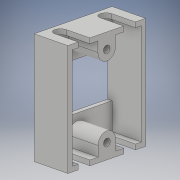
# Autodesk Inventor part: ssr-cover
Saved by Autodesk Inventor 2018 (Build 220112000, 112)
## iProperties
Created: 2020-01-09
Part Number: ssr-cover
Material: Generic
Document SubType Name: Modeling
Designer: Vinnie Caprarola
Density: 1 g/cm^3
Appearance: Default
Author: Vinnie Caprarola
Autodesk Inventor part; units mm, degrees
ref_plane "YZ Plane" through (0, 0, 0) normal (1, 0, 0) x (0, 1, 0)
sketch "Sketch1" plane through (0, 0, 0) normal (0, 0, 1) x (1, 0, 0)
  line L0 (0, 0) -> (45, 0)
  line L1 (45, 0) -> (45, 58)
  line L2 (45, 58) -> (0, 58)
  line L3 (0, 58) -> (0, 0)
  circle A0 centre (22.5, 53) radius 2.75
  circle A1 centre (22.5, 5) radius 2.75
  line L4 (19.75, 58) -> (19.75, 53)
  line L5 (25.25, 58) -> (25.25, 53)
  line L6 (0, 42) -> (45, 42)
  line L7 (45, 42) -> (45, 16)
  line L8 (45, 16) -> (0, 16)
  line L9 (0, 16) -> (0, 42)
  circle A2 centre (22.5, 53) radius 6
  circle A3 centre (22.5, 5) radius 6
  line L10 (16.5, 5) -> (16.5, -1)
  line L11 (28.5, 5) -> (28.5, -1)
  line L12 (16.5, 53) -> (16.5, 59)
  line L13 (28.5, 53) -> (28.5, 59)
  line L14 (-1, 59) -> (46, 59)
  line L15 (46, 59) -> (46, -1)
  line L16 (46, -1) -> (-1, -1)
  line L17 (-1, -1) -> (-1, 59)
  line L18 (49, 62) -> (-4, 62)
  line L19 (-4, 62) -> (-4, -4)
  line L20 (-4, -4) -> (49, -4)
  line L21 (49, -4) -> (49, 62)
  line L22 (28.5, 59) -> (16.5, 59)
  line L23 (28.5, -1) -> (16.5, -1)
  point P0 (22.5, 58)
  dimension "d0" = 45
  dimension "d1" = 58
  dimension "d2" = 5.5
  dimension "d3" = 5.5
  dimension "d4" = 5
  dimension "d5" = 5
  dimension "d6" = 26
  dimension "d7" = 16
  dimension "d8" = 12
  dimension "d9" = 12
  dimension "d10" = 1
  dimension "d11" = 3
  constraints: 48 end point, 10 parallel, 10 point on line, 6 perpendicular, 6 point on circle, 4 centre point, 4 tangent, 2 coincident, 2 horizontal, 2 vertical alignment, 1 collinear, 1 midpoint, 1 vertical, 6 other
  measures "d0" distance of L1.end L2.end
  measures "d1" distance of L0.end L1.end
  measures "d2" diameter of A0
  measures "d3" diameter of A1
  measures "d4" distance from line of A1.centre L0
  measures "d5" distance from line of A0.centre L2
  measures "d6" distance between parallel lines of L8 L6
  measures "d7" distance between parallel lines of L6 L2
  measures "d8" diameter of A2
  measures "d9" diameter of A3
  measures "d10" distance between parallel lines of L2 L14
  measures "d11" distance between parallel lines of L14 L18
extrude "Extrusion1" add sketch "Sketch1" along normal blind 10 contours L21 L20 L19 L18
sketch "Sketch2" plane through (0, 0, 10) normal (0, 0, 1) x (1, 0, 0)
  line L0 (-1, 59) -> (46, 59) projected
  line L1 (46, 59) -> (46, -1) projected
  line L2 (-1, 59) -> (46, 59)
  line L3 (46, 59) -> (46, 43)
  line L4 (46, 43) -> (-1, 43)
  line L5 (-1, 43) -> (-1, 59)
  line L6 (-1, -1) -> (-1, 59) projected
  line L7 (46, -1) -> (-1, -1)
  line L8 (-1, -1) -> (-1, 15)
  line L9 (-1, 15) -> (46, 15)
  line L10 (46, 15) -> (46, -1)
  point P0 (0, 0)
  dimension "d14" = 16
  dimension "d15" = 16
  constraints: 16 end point, 4 parallel, 2 horizontal, 2 perpendicular, 2 point on line
  measures "d14" distance of L2.end L3.end
  measures "d15" distance of L7.end L8.end
extrude "Extrusion2" add sketch "Sketch2" against normal blind 3 contours L0 L1 L4 L5 | L9 L1 L7 L6
sketch "Sketch3" plane through (0, 0, 0) normal (0, 0, -1) x (-1, 0, 0)
  arc A0 (-28.5, 53) -> (-16.5, 53) centre (-22.5, 53) ccw
  line L0 (-46, 59) -> (1, 59) projected
  line L1 (-28.5, 59) -> (-28.5, 53)
  line L2 (-16.5, 59) -> (-16.5, 53)
  line L3 (-16.5, 59) -> (-28.5, 59)
  point P0 (0, 0)
  dimension "d18" = 12
  constraints: 6 end point, 2 perpendicular, 2 point on circle, 2 point on line, 1 centre point, 1 coincident, 1 parallel
  measures "d18" diameter of A0
extrude "Extrusion3" add sketch "Sketch3" against normal up to surface (7 mm away)
ref_plane "Work Plane1" through (-4, 29, 0) normal (0, 1, 0) x (1, 0, 0)
mirror "Mirror1" about plane through (-4, 29, 0) normal (0, 1, 0) of "Extrusion3"
thicken "Thicken1" operation add thickness 13 both sides no extend neighbours yes toward (0, 0, -1) faces at (48, 39, 0)
sketch "Sketch4" plane through (-4, 62, 10) normal (0, 1, 0) x (1, 0, 0)
  line L0 (3, 3) -> (3, 0) projected
  line L1 (3, 0) -> (3, 3) projected
  line L2 (3, 23) -> (3, 3) projected
  line L3 (3, 23) -> (3, 3) projected
  line L4 (50, 0) -> (50, 3) projected
  line L5 (50, 23) -> (50, 3) projected
  line L6 (50, 23) -> (50, 3) projected
  line L7 (50, 3) -> (50, 0) projected
  line L8 (20.5, 3) -> (32.5, 3) projected
  line L9 (50, 3) -> (32.5, 3) projected
  line L10 (50, 3) -> (3, 3) projected
  line L11 (20.5, 3) -> (3, 3) projected
  line L12 (32.5, 23) -> (32.5, 3) projected
  line L13 (32.5, 23) -> (32.5, 3) projected
  line L14 (20.5, 23) -> (20.5, 3) projected
  line L15 (20.5, 3) -> (20.5, 23) projected
  line L16 (53, 23) -> (0, 23) projected
  line L17 (42, 23) -> (42, 7) construction
  line L18 (38, 23) -> (38, 7)
  line L19 (46, 7) -> (46, 23)
  arc A0 (46, 23) -> (38, 23) centre (42, 23) ccw
  arc A1 (38, 7) -> (46, 7) centre (42, 7) ccw
  point P0 (4, 10)
  point P1 (42, 15)
  dimension "d23" = 4
  dimension "d24" = 8
  dimension "d25" = 16
  constraints: 8 end point, 4 point on circle, 4 tangent, 2 centre point, 1 midpoint, 1 parallel, 1 vertical, 2 other
  measures "d23" distance between parallel lines of L5 L19
  measures "d24" distance between parallel lines of L18 L19
extrude "Extrusion4" cut sketch "Sketch4" against normal through all contours L16 L19 A1 L18
ref_plane "Work Plane2" through (22.5, -4, 10) normal (1, 0, 0) x (0, 0, -1)
mirror "Mirror2" about plane through (22.5, -4, 10) normal (1, 0, 0) of "Extrusion4"
hole "Hole1" at (22.5, 53, 10) direction (0, 0, -1) diameter 4.5 end through all counterbore diameter 8 counterbore depth 4 clearance for "Socket Head Cap Screw" size "M4" standard "Ansi Metric M Profile"
mirror "Mirror3" about plane through (-4, 29, 0) normal (0, 1, 0) of "Hole1"
body "Solid1"
